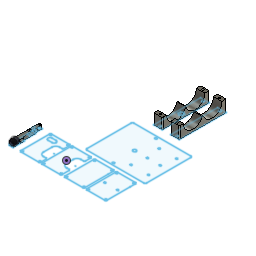
FTR102_R2_v4 (Autodesk Fusion 360 design; units mm, degrees)
Autodesk Fusion 360 part; units mm, degrees
sketch "スケッチ1" plane through (0, 0, 0) normal (0, 0, 1) x (1, 0, 0)
  line L0 (21.5, 36) -> (-21.5, 36)
  line L1 (-23.5, 34) -> (-23.5, -34)
  line L2 (-21.5, -36) -> (21.5, -36)
  circle A0 centre (-20.5, -33) radius 1.6
  circle A1 centre (20.5, -33) radius 1.6
  arc A2 (-23.5, -34) -> (-21.5, -36) centre (-21.5, -34) ccw
  arc A3 (-21.5, 36) -> (-23.5, 34) centre (-21.5, 34) ccw
  arc A4 (23.5, 34) -> (21.5, 36) centre (21.5, 34) ccw
  arc A5 (21.5, -36) -> (23.5, -34) centre (21.5, -34) ccw
  line L3 (21.5, -15) -> (16, -15)
  line L4 (23.5, -34) -> (23.5, -17)
  arc A6 (15.5314, -14.9843) -> (16, -15) centre (16, -8) ccw
  arc A7 (23.5, -17) -> (21.5, -15) centre (21.5, -17) ccw
  arc A8 (21.5, -1) -> (22.3523, -0.8093) centre (21.5, 1) ccw
  line L5 (6, -6) -> (6, 10)
  line L6 (15, 19) -> (21.5, 19)
  line L7 (23.5, 21) -> (23.5, 34)
  arc A9 (6, -6) -> (15.5314, -14.9843) centre (15, -6) ccw
  arc A10 (15, 19) -> (6, 10) centre (15, 10) ccw
  arc A11 (21.5, 19) -> (23.5, 21) centre (21.5, 21) ccw
  line L8 (30, 34) -> (30, -34)
  line L9 (32, -36) -> (75, -36)
  arc A12 (32, 36) -> (30, 34) centre (32, 34) ccw
  arc A13 (30, -34) -> (32, -36) centre (32, -34) ccw
  circle A14 centre (33, -33) radius 1.6
  line L10 (77, 21) -> (77, 34)
  arc A15 (77, 34) -> (75, 36) centre (75, 34) ccw
  line L11 (77, -34) -> (77, 21)
  circle A16 centre (74, -33) radius 1.6
  line L12 (75, 36) -> (32, 36)
  arc A17 (75, -36) -> (77, -34) centre (75, -34) ccw
  line L13 (81.5, 34) -> (81.5, -34)
  arc A18 (126.5, -36) -> (128.5, -34) centre (126.5, -34) ccw
  line L14 (83.5, -36) -> (126.5, -36)
  arc A19 (81.5, -34) -> (83.5, -36) centre (83.5, -34) ccw
  line L15 (126.5, 36) -> (83.5, 36)
  arc A20 (128.5, 34) -> (126.5, 36) centre (126.5, 34) ccw
  circle A21 centre (125.5, -33) radius 1.6
  arc A22 (83.5, 36) -> (81.5, 34) centre (83.5, 34) ccw
  circle A23 centre (84.5, -33) radius 1.6
  line L16 (128.5, 21) -> (128.5, 34)
  line L17 (128.5, -34) -> (128.5, 21)
  circle A24 centre (90, 0) radius 1.6
  circle A25 centre (120, 0) radius 1.6
  arc A26 (-73.5, -34) -> (-71.5, -36) centre (-71.5, -34) ccw
  circle A27 centre (-70.5, -33) radius 1.6
  line L18 (-73.5, 34) -> (-73.5, -34)
  arc A28 (-71.5, 36) -> (-73.5, 34) centre (-71.5, 34) ccw
  line L19 (-35, 19) -> (-28.5, 19)
  arc A29 (-28.5, 19) -> (-26.5, 21) centre (-28.5, 21) ccw
  line L20 (-44, -10) -> (-44, 10)
  circle A30 centre (-29.5, -33) radius 1.6
  arc A31 (-28.5, -36) -> (-26.5, -34) centre (-28.5, -34) ccw
  line L21 (-26.5, -34) -> (-26.5, -21)
  arc A32 (-26.5, 34) -> (-28.5, 36) centre (-28.5, 34) ccw
  arc A33 (-28.5, -1) -> (-27.6477, -0.8093) centre (-28.5, 1) ccw
  circle A34 centre (-29.5, 33) radius 1.6
  line L22 (-26.5, 21) -> (-26.5, 34)
  arc A35 (-35, 19) -> (-44, 10) centre (-35, 10) ccw
  line L23 (-71.5, -36) -> (-28.5, -36)
  line L24 (-28.5, 36) -> (-71.5, 36)
  line L25 (-62.5, 28.5) -> (-53, 28.5)
  line L26 (-48.5, 24.0011) -> (-48.5, 23.9989)
  line L27 (-53, 19.5) -> (-62.5, 19.5)
  arc A36 (-62.5, 28.5) -> (-62.5, 19.5) centre (-62.5, 24) ccw
  arc A37 (-53.0011, 19.5) -> (-53, 28.5) centre (-53, 24) ccw
  circle A38 centre (-20.5, 33) radius 1.6
  circle A39 centre (20.5, 33) radius 1.6
  circle A40 centre (-70.5, 33) radius 1.6
  circle A41 centre (33, 33) radius 1.6
  circle A42 centre (74, 33) radius 1.6
  circle A43 centre (84.5, 33) radius 1.6
  circle A44 centre (125.5, 33) radius 1.6
  circle A45 centre (-97, 33) radius 1.6
  arc A46 (-100, -34) -> (-98, -36) centre (-98, -34) ccw
  circle A47 centre (-97, -33) radius 1.6
  arc A48 (-98, 36) -> (-100, 34) centre (-98, 34) ccw
  line L28 (-93, 36) -> (-93, 18)
  line L29 (-93, -36) -> (-98, -36)
  line L30 (-98, 36) -> (-93, 36)
  line L31 (-95, 25.5) -> (-100, 25.5)
  line L32 (-100, 19.5) -> (-95, 19.5)
  line L33 (-95, 19.5) -> (-95, 25.5)
  line L34 (-100, 34) -> (-100, 25.5)
  line L35 (-99, 13) -> (-94, 13)
  line L36 (-94, 7) -> (-99, 7)
  line L37 (-99, 7) -> (-99, 13)
  line L38 (-94, 7) -> (-94, 13)
  line L39 (-93, -36) -> (-91, -36)
  line L40 (-91, -10) -> (-91, 18)
  line L41 (-93, 18) -> (-91, 18)
  line L42 (-89, -10) -> (-91, -10)
  line L43 (-91, -36) -> (-89, -36)
  line L44 (-89, -36) -> (-89, -10)
  line L45 (-91, -19.5) -> (-100, -19.5)
  line L46 (-100, -25.5) -> (-91, -25.5)
  line L47 (-91, -25.5) -> (-91, -19.5)
  line L48 (-100, 19.5) -> (-100, -19.5)
  line L49 (-100, -25.5) -> (-100, -34)
  line L50 (-100, -25.5) -> (-100, -19.5)
  line L51 (-100, 19.5) -> (-100, 25.5)
  arc A49 (-44, -10) -> (-35, -19) centre (-35, -10) ccw
  line L52 (-35, -19) -> (-28.5, -19)
  arc A50 (-26.5, -21) -> (-28.5, -19) centre (-28.5, -21) ccw
  circle A51 centre (90, 100) radius 1.6
  circle A52 centre (125.5, 133) radius 1.6
  circle A53 centre (84.5, 133) radius 1.6
  circle A54 centre (84.5, 67) radius 1.6
  circle A55 centre (120, 100) radius 1.6
  circle A56 centre (125.5, 67) radius 1.6
  line L53 (3, 45) -> (137, 45)
  line L54 (140, 48) -> (140, 152)
  line L55 (137, 155) -> (3, 155)
  line L56 (0, 152) -> (0, 48)
  circle A57 centre (60, 50) radius 2.1
  circle A58 centre (60, 150) radius 2.1
  arc A59 (0, 48) -> (3, 45) centre (3, 48) ccw
  arc A60 (3, 155) -> (0, 152) centre (3, 152) ccw
  arc A61 (140, 152) -> (137, 155) centre (137, 152) ccw
  arc A62 (137, 45) -> (140, 48) centre (137, 48) ccw
  circle A63 centre (40, 180) radius 2.2
  line L57 (30, 285) -> (30, 175)
  line L58 (30, 175) -> (50, 175)
  line L59 (50, 285) -> (30, 285)
  circle A64 centre (40, 280) radius 2.2
  line L60 (50, 175) -> (50, 285)
  line L61 (39.9738, 235.8889) -> (34.8869, 232.9218)
  line L62 (34.8869, 232.9218) -> (34.9132, 227.0328)
  line L63 (34.9132, 227.0328) -> (40.0262, 224.1111)
  line L64 (40.0262, 224.1111) -> (45.1131, 227.0783)
  line L65 (45.1131, 227.0783) -> (45.0868, 232.9672)
  line L66 (45.0868, 232.9672) -> (39.9738, 235.8889)
  circle A65 centre (40, 230) radius 3.5
  line L67 (70, 175) -> (90, 175)
  line L68 (90, 175) -> (90, 285)
  line L69 (70, 285) -> (70, 175)
  line L70 (90, 285) -> (70, 285)
  circle A66 centre (80, 280) radius 2.2
  circle A67 centre (80, 180) radius 2.2
  circle A68 centre (60, 100) radius 3.5
  point P0 (-25, -37.5)
  point P1 (-25, 37.5)
  point P2 (25, 37.5)
  point P3 (-23.5, 36)
  point P4 (-23.5, -36)
  point P5 (23.5, -36)
  point P6 (80, 37.5)
  point P7 (53.5, 0)
  point P8 (53.5, 0)
  point P9 (53.5, 0)
  point P10 (28.5, -37.5)
  point P11 (30, 37.485)
  point P12 (30, 36)
  point P13 (30, -36)
  point P14 (53.5, 0)
  point P15 (77, -36)
  point P16 (81.5, -36)
  point P17 (128.5, -36)
  point P18 (105, 0)
  point P19 (80, -37.5)
  point P20 (81.5, 36)
  point P21 (105, 0)
  point P22 (105, 0)
  point P23 (105, 0)
  point P24 (80, 37.5)
  point P25 (130, 37.5)
  point P26 (105, 0)
  point P27 (-73.5, -36)
  point P28 (-26.5, -36)
  point P29 (-73.5, 36)
  point P30 (-75, -37.5)
  point P31 (-25, 37.5)
  point P32 (-75, 37.5)
  point P33 (-21.5, 34)
  point P34 (21.5, 34)
  point P35 (-71.5, 34)
  point P36 (-28.5, 34)
  point P37 (32, 34)
  point P38 (75, 34)
  point P39 (32, 34)
  point P40 (75, 34)
  point P41 (83.5, 34)
  point P42 (126.5, 34)
  point P43 (83.5, 34)
  point P44 (126.5, 34)
  point P45 (-100, -36)
  point P46 (-101.5, -37.5)
  point P47 (-100, 36)
  point P48 (-101.5, 37.5)
  point P49 (-98, 34)
  point P50 (126.5, 134)
  point P51 (83.5, 134)
  point P52 (105, 100)
  point P53 (128.5, 64)
  point P54 (126.5, 134)
  point P55 (81.5, 64)
  point P56 (83.5, 134)
  point P57 (80, 137.5)
  point P58 (105, 100)
  point P59 (80, 62.5)
  point P60 (81.5, 136)
  point P61 (105, 100)
  point P62 (80, 137.5)
  point P63 (130, 137.5)
  point P64 (105, 100)
  point P65 (105, 100)
  point P66 (65, 100)
  point P67 (50, 45)
  point P68 (30, 175)
  point P69 (40, 230)
  point P70 (70, 175)
  dimension "d3" = 50
  dimension "d4" = 75
  dimension "d36" = 47
  dimension "d37" = 72
  dimension "d38" = 3.2
  dimension "d40" = 2
  dimension "d43" = 14
  dimension "d44" = 2
  dimension "d48" = 18
  dimension "d49" = 2
  dimension "d50" = 50
  dimension "d51" = 75
  dimension "d52" = 47
  dimension "d53" = 72
  dimension "d54" = 3.2
  dimension "d56" = 2
  dimension "d61" = 50
  dimension "d62" = 75
  dimension "d63" = 47
  dimension "d64" = 72
  dimension "d65" = 3.2
  dimension "d67" = 2
  dimension "d69" = 3.2
  dimension "d70" = 3.2
  dimension "d71" = 50
  dimension "d72" = 75
  dimension "d73" = 47
  dimension "d74" = 72
  dimension "d75" = 3.2
  dimension "d77" = 2
  dimension "d81" = 2
  dimension "d82" = 9
  dimension "d83" = 9
  dimension "d86" = 3.2
  dimension "d87" = 3.2
  dimension "d88" = 3.2
  dimension "d89" = 3.2
  dimension "d90" = 75
  dimension "d91" = 72
  dimension "d92" = 3.2
  dimension "d94" = 2
  dimension "d95" = 3.2
  dimension "d96" = 6
  dimension "d113" = 50
  dimension "d114" = 75
  dimension "d115" = 47
  dimension "d116" = 72
  dimension "d117" = 3.2
  dimension "d119" = 3.2
  dimension "d120" = 3.2
  dimension "d121" = 3.2
  dimension "d128" = 4.2
  dimension "d129" = 4.2
  dimension "d130" = 3
  dimension "d131" = 20
  dimension "d132" = 110
  dimension "d133" = 4.4
  dimension "d134" = 4.4
  dimension "d136" = 5.1
  dimension "d146" = 7
  dimension "d151" = 20
  dimension "d152" = 110
  dimension "d153" = 4.4
  dimension "d154" = 4.4
  dimension "d165" = 7
  constraint horizontal L0
  constraint perpendicular L0 L1
  constraint parallel L0 L2
  constraint parallel L1 L4
  constraint coincident P4 L2
  constraint coincident P4 L1
  constraint tangent L2 A2
  constraint tangent L1 A2
  constraint coincident P3 L0
  constraint coincident P3 L1
  constraint tangent L0 A3
  constraint tangent L1 A3
  constraint equal A2 A3
  constraint tangent L0 A4
  constraint tangent A4 L4
  constraint equal A2 A4
  constraint coincident P5 L2
  constraint coincident P5 L4
  constraint tangent L2 A5
  constraint tangent A5 L4
  constraint equal A2 A5
  constraint tangent L3 A6
  constraint tangent L3 A7
  constraint tangent L4 A7
  constraint equal A7 A8
  constraint vertical L5
  constraint horizontal L6
  constraint tangent L7 A11
  constraint tangent L6 A11
  constraint coincident P14 P9
  constraint horizontal L12
  constraint perpendicular L8 L12
  constraint parallel L9 L12
  constraint parallel L8 L11
  constraint coincident P13 L9
  constraint coincident P13 L8
  constraint tangent L9 A13
  constraint tangent L8 A13
  constraint coincident P12 L12
  constraint coincident P12 L8
  constraint tangent A12 L12
  constraint tangent L8 A12
  constraint equal A12 A13
  constraint tangent A15 L12
  constraint tangent A15 L11
  constraint equal A13 A15
  constraint coincident P15 L9
  constraint coincident P15 L11
  constraint tangent L9 A17
  constraint tangent L11 A17
  constraint equal A13 A17
  constraint coincident P26 P23
  constraint horizontal L15
  constraint perpendicular L13 L15
  constraint parallel L14 L15
  constraint parallel L13 L17
  constraint coincident P16 L14
  constraint coincident P16 L13
  constraint tangent L14 A19
  constraint tangent L13 A19
  constraint coincident P20 L15
  constraint coincident P20 L13
  constraint tangent L15 A22
  constraint tangent L13 A22
  constraint equal A19 A22
  constraint tangent L15 A20
  constraint tangent A20 L17
  constraint equal A19 A20
  constraint coincident P17 L14
  constraint coincident P17 L17
  constraint tangent A18 L14
  constraint tangent A18 L17
  constraint equal A18 A19
  constraint horizontal L24
  constraint perpendicular L18 L24
  constraint parallel L23 L24
  constraint parallel L18 L21
  constraint coincident P27 L23
  constraint coincident P27 L18
  constraint tangent A26 L23
  constraint tangent A26 L18
  constraint coincident P29 L24
  constraint coincident P29 L18
  constraint tangent A28 L24
  constraint tangent L18 A28
  constraint equal A26 A28
  constraint tangent A32 L24
  constraint tangent L21 A32
  constraint equal A26 A32
  constraint coincident P28 L23
  constraint coincident P28 L21
  constraint tangent A31 L23
  constraint tangent A31 L21
  constraint equal A26 A31
  constraint vertical L20
  constraint horizontal L19
  constraint tangent A29 L22
  constraint tangent L19 A29
  constraint horizontal L25
  constraint perpendicular L25 L26
  constraint parallel L25 L27
  constraint coincident L27.start A37
  constraint coincident L26.end A37
  constraint coincident L26.start A37
  constraint coincident L27 A37.start
  constraint coincident P45 L34
  constraint tangent A46 L34
  constraint coincident P47 L34
  constraint tangent A48 L34
  constraint equal A46 A48
  constraint vertical L28
  constraint tangent A46 L29
  constraint horizontal L31
  constraint horizontal L32
  constraint vertical L33
  constraint coincident L32.start L34
  constraint collinear L34 L48
  constraint horizontal L35
  constraint horizontal L36
  constraint vertical L37
  constraint perpendicular L35 L38
  constraint perpendicular L28 L39
  constraint perpendicular L29 L40
  constraint perpendicular L40 L41
  constraint horizontal L42
  constraint horizontal L43
  constraint vertical L44
  constraint horizontal L45
  constraint horizontal L46
  constraint vertical L47
  constraint collinear L48 L49
  constraint perpendicular L45 L50
  constraint perpendicular L31 L51
  constraint coincident L21.end A50
  constraint tangent L21 A50
  constraint coincident P65 P64
  constraint horizontal L53
  constraint vertical L54
  constraint horizontal L55
  constraint vertical L56
  constraint tangent L53 A59
  constraint tangent L56 A59
  constraint tangent L55 A60
  constraint tangent L56 A60
  constraint equal A59 A60
  constraint tangent L54 A61
  constraint tangent L55 A61
  constraint equal A59 A61
  constraint tangent L53 A62
  constraint tangent L54 A62
  constraint equal A59 A62
  constraint horizontal L59
  constraint perpendicular L57 L59
  constraint parallel L58 L59
  constraint parallel L57 L60
  constraint coincident P68 L57.end
  constraint coincident P69 A65.centre
  constraint horizontal L70
  constraint perpendicular L69 L70
  constraint parallel L67 L70
  constraint parallel L68 L69
  constraint coincident P70 L67.start
  measures "d3" distance of P31 P2
  measures "d4" distance of P0 P31
  measures "d36" distance of P4 P5
  measures "d37" distance of P3 P4
  measures "d38" diameter of A0
  measures "d40" radius of A2
  measures "d43" diameter of A6
  measures "d44" radius of A7
  measures "d48" diameter of A9
  measures "d49" radius of A11
  measures "d50" distance of P24 P11
  measures "d51" distance of P10 P11
  measures "d52" distance of P13 P15
  measures "d53" distance of P12 P13
  measures "d54" diameter of A14
  measures "d56" radius of A13
  measures "d61" distance of P24 P25
  measures "d62" distance of P19 P24
  measures "d63" distance of P16 P17
  measures "d64" distance of P16 P20
  measures "d65" diameter of A23
  measures "d67" radius of A19
  measures "d69" diameter of A24
  measures "d70" diameter of A25
  measures "d71" distance of P31 P32
  measures "d72" distance of P30 P32
  measures "d73" distance of P27 P28
  measures "d74" distance of P27 P29
  measures "d75" diameter of A27
  measures "d77" radius of A26
  measures "d81" radius of A29
  measures "d82" diameter of A37
  measures "d83" diameter of A36
  measures "d86" diameter of A38
  measures "d87" diameter of A40
  measures "d88" diameter of A41
  measures "d89" diameter of A43
  measures "d90" distance of P46 P48
  measures "d91" distance of P45 P47
  measures "d92" diameter of A47
  measures "d94" radius of A46
  measures "d95" diameter of A45
  measures "d96" distance of L45.start L46.end
  measures "d113" distance of P62 P63
  measures "d114" distance of P59 P62
  measures "d115" distance of P53 P55
  measures "d116" distance of P55 P60
  measures "d117" diameter of A54
  measures "d119" diameter of A51
  measures "d120" diameter of A55
  measures "d121" diameter of A53
  measures "d128" diameter of A57
  measures "d129" diameter of A58
  measures "d130" radius of A59
  measures "d131" distance of P68 L58.end
  measures "d132" distance of L57.start P68
  measures "d133" diameter of A63
  measures "d134" diameter of A64
  measures "d136" distance of P69 L66
  measures "d146" diameter of A65
  measures "d151" distance of P70 L67.end
  measures "d152" distance of P70 L69.start
  measures "d153" diameter of A67
  measures "d154" diameter of A66
  measures "d165" diameter of A68
extrude "押し出し1" add sketch "スケッチ1" along normal blind 8 contours A46 A48 L28 L29 L30 L31 L32 L33 L34 L39 L40 L41 L42 L43 L44 L45 L46 L47 L48 L49 | L45 L46 L47 L50 | L31 L32 L33 L51 | L35 L36 L37 L38 makes body 1
sketch "スケッチ2" plane through (-100, 0, 0) normal (-1, 0, 0) x (0, -1, 0)
  line L0 (-34, 0) -> (34, 0)
  line L1 (34, 0) -> (34, 8)
  line L2 (34, 8) -> (-34, 8)
  line L3 (-34, 8) -> (-34, 0)
  line L4 (-19.5, 6) -> (-25.5, 6)
  line L5 (-25.5, 6) -> (-25.5, 0)
  line L6 (-25.5, 0) -> (-19.5, 0)
  line L7 (-19.5, 0) -> (-19.5, 6)
  line L8 (19.5, 0) -> (19.5, 3)
  line L9 (25.5, 0) -> (25.5, 3.0005)
  arc A0 (25.5, 2.9995) -> (19.5, 3) centre (22.5, 3) ccw
  line L10 (19.5, 0) -> (25.5, 0)
  point P0 (19.5, 0)
  point P1 (25.5, 0)
  dimension "d99" = 6
  dimension "d100" = 6
  constraint horizontal L4
  constraint vertical L5
  constraint horizontal L6
  constraint vertical L7
  constraint coincident P0 L8.start
  constraint perpendicular L0 L8
  constraint coincident P1 L9.start
  constraint perpendicular L0 L9
  constraint coincident L9.end A0
  constraint coincident L9 A0.start
  measures "d99" diameter of A0
  measures "d100" distance of L4.start L4.end
extrude "押し出し2" cut sketch "スケッチ2" against normal blind 5.5 contours L0 L4 L5 L6 L7 bodies 1
extrude "押し出し3" cut sketch "スケッチ2" against normal blind 11 contours L0 L8 L9 A0 L10 bodies 1
extrude "押し出し4" cut sketch "スケッチ1" along normal blind 8 contours L35 L36 L37 L38 bodies 1
fillet "フィレット1" radius 1 1 edges at (-93, 36, 4) on bodies 1
fillet "フィレット2" radius 1 3 edges at (-89, -36, 4) (-89, -10, 4) (-91, -10, 4) on bodies 1
fillet "フィレット3" radius 1 2 edges at (-91, 18, 4) (-93, 18, 4) on bodies 1
extrude "押し出し5" add sketch "スケッチ1" along normal blind 24.5 separate body contours L57 L58 L59 L60 makes body 2
sketch "スケッチ3" plane through (50, 0, 0) normal (1, 0, 0) x (0, 1, 0)
  line L0 (175, 0) -> (285, 0)
  line L1 (285, 0) -> (285, 24.5)
  line L2 (285, 24.5) -> (175, 24.5)
  line L3 (175, 24.5) -> (175, 0)
  arc A0 (185, 24.5) -> (229.5454, 20) centre (207.5, 24.5) ccw
  arc A1 (230.4546, 20) -> (275, 24.5) centre (252.5, 24.5) ccw
  line L4 (229.5454, 20) -> (230.4546, 20)
  point P0 (230, 15)
  dimension "d140" = 45
  dimension "d141" = 45
  constraint coincident L2 A0.centre
  constraint coincident L2 A1.centre
  constraint coincident L2 A0.start
  constraint coincident L2 A1.end
  constraint horizontal L4
  measures "d140" diameter of A0
  measures "d141" diameter of A1
extrude "押し出し6" add sketch "スケッチ1" along normal blind 24.5 contours L61 L62 L63 L64 L65 L66 | A65 bodies 2
extrude "押し出し7" cut sketch "スケッチ1" along normal blind 5.4 contours L61 L62 L63 L64 L65 L66 | A65 bodies 2
extrude "押し出し8" cut sketch "スケッチ1" along normal blind 10 contours A65 bodies 2
extrude "押し出し9" cut sketch "スケッチ3" against normal blind 20 contours L2 A0 A1 L4 bodies 2
extrude "押し出し10" add sketch "スケッチ1" along normal blind 27.5 separate body contours L67 L68 L69 L70 makes body 3
sketch "スケッチ4" plane through (90, 0, 0) normal (1, 0, 0) x (0, 1, 0)
  line L0 (175, 0) -> (285, 0)
  line L1 (285, 0) -> (285, 27.5)
  line L2 (285, 27.5) -> (175, 27.5)
  line L3 (175, 27.5) -> (175, 0)
  line L4 (228.7132, 20) -> (231.2868, 20)
  arc A0 (185, 27.5) -> (228.7132, 20) centre (207.5, 27.5) ccw
  arc A1 (231.2868, 20) -> (275, 27.5) centre (252.5, 27.5) ccw
  point P0 (230, 14.9867)
  dimension "d161" = 45
  dimension "d162" = 45
  constraint coincident L2 A0.centre
  constraint coincident L2 A1.centre
  constraint horizontal L4
  constraint coincident L2 A0.start
  constraint coincident L2 A1.end
  measures "d161" diameter of A0
  measures "d162" diameter of A1
extrude "押し出し11" cut sketch "スケッチ4" against normal blind 20 contours L2 L4 A0 A1 bodies 3
fillet "フィレット4" radius 2 4 edges at (30, 175, 12.25) (50, 175, 12.25) (70, 175, 13.75) (90, 175, 13.75) on bodies 2 3
fillet "フィレット5" radius 2 4 edges at (50, 285, 12.25) (30, 285, 12.25) (90, 285, 13.75) (70, 285, 13.75) on bodies 2 3
